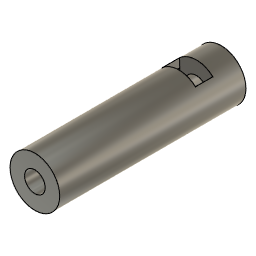
shaft_sa4_sa5_servo v1 (Autodesk Fusion 360 design; units mm, degrees)
Autodesk Fusion 360 part; units mm, degrees
sketch "Sketch1" plane through (0, 0, 0) normal (0, 1, 0) x (1, 0, 0)
  circle A0 centre (0, 0) radius 6
  dimension "d1" = 12
  constraint coincident A0.centre origin
  measures "d1" diameter of A0
extrude "Extrude1" add sketch "Sketch1" along normal blind 45
sketch "Sketch2" plane through (0, 0, 0) normal (0, -1, 0) x (1, 0, 0)
  circle A0 centre (0, 0) radius 6
  circle A1 centre (0, 0) radius 1.6031
  circle A2 centre (0, 0) radius 2.5
  circle A3 centre (0, 0) radius 2
  dimension "d4" = 5
  dimension "d5" = 4
  constraint coincident A0.centre A1.centre
  constraint concentric A1 A2
  constraint concentric A1 A3
  measures "d4" diameter of A2
  measures "d5" diameter of A3
extrude "Extrude2" cut sketch "Sketch2" against normal blind 5.5 contours A2
extrude "Extrude3" cut 1 faces at (1.1392, 0, 0.5006) along direction (0, 1, 0) blind 71
sketch "Sketch3" plane through (0, 45, 0) normal (0, 1, 0) x (-1, 0, 0)
  circle A0 centre (0, 0) radius 2
  circle A1 centre (0, 0) radius 6
  circle A2 centre (0, 0) radius 2.75
  dimension "d10" = 5.5
  constraint coincident A0.centre A1.centre
  measures "d10" diameter of A2
extrude "Extrude4" cut sketch "Sketch3" against normal blind 24 contours A2
ref_plane "WorkPlane1" through (0, 39, 0) normal (0, 1, 0) x (1, 0, 0)
sketch "Sketch4" plane through (0, 39, 0) normal (0, 1, 0) x (1, 0, 0)
  line L0 (4, 2.3094) -> (0, 4.6188)
  line L1 (0, 4.6188) -> (-4, 2.3094)
  line L2 (-4, 2.3094) -> (-4, -2.3094)
  line L3 (-4, -2.3094) -> (0, -4.6188)
  line L4 (0, -4.6188) -> (4, -2.3094)
  line L5 (4, -2.3094) -> (4, 2.3094)
  line L6 (4, -2.3094) -> (4, -7)
  line L7 (4, -7) -> (-4.1244, -7)
  line L8 (-4.1244, -7) -> (-4, -2.3094)
  dimension "d14" = 4
  constraint parallel L5 L6
  constraint perpendicular L6 L7
  measures "d14" distance of origin L5
extrude "Extrude5" cut sketch "Sketch4" against normal blind 4.2
